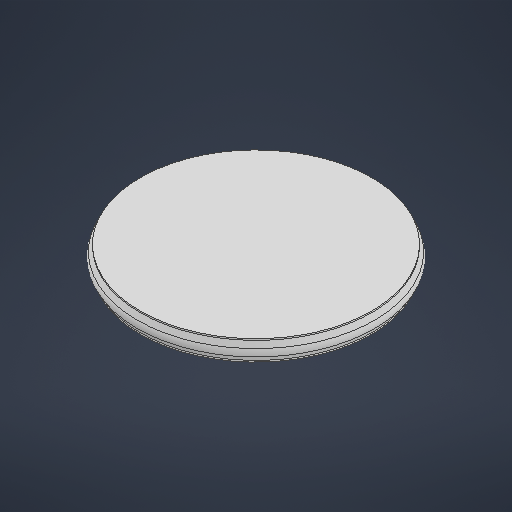
# Autodesk Inventor part: Game-Piece
Saved by Autodesk Inventor 2025 (Build 290162010, 162A)
## iProperties
Created: 2025-10-23
Part Number: Game-Piece
Material: Generic
Document SubType Name: Modeling
Designer: FizzyApple12
Density: 1 g/cm^3
Appearance: Default
Author: FizzyApple12
Autodesk Inventor part; units mm, degrees
ref_plane "YZ Plane" through (0, 0, 0) normal (1, 0, 0) x (0, 1, 0)
ref_plane "XZ Plane" through (0, 0, 0) normal (0, 1, 0) x (-1, 0, 0)
ref_plane "XY Plane" through (0, 0, 0) normal (0, 0, 1) x (1, 0, 0)
sketch "Sketch1" plane through (0, 0, 0) normal (1, 0, 0) x (0, 1, 0)
  line L0 (2.8, 16) -> (0, 16)
  line L1 (0, 16) -> (0, -16)
  line L2 (0, -16) -> (2.8, -16)
  line L3 (2.8, -16) -> (2.8, 16)
  line L4 (2.4, 12.7) -> (0.4, 12.7)
  line L5 (0.4, 12.7) -> (0.4, -12.7)
  line L6 (0.4, -12.7) -> (2.4, -12.7)
  line L7 (2.4, -12.7) -> (2.4, 12.7)
  line L8 (0, 0) -> (2.8, 0)
  line L9 (0.2, 16) -> (1.4, 16.6928)
  line L10 (1.4, 16.6928) -> (2.6, 16)
  line L11 (1.4, 16.6928) -> (1.4, 12.7) construction
  point P0 (0.4, 0)
  point P1 (2.4, 0)
  dimension "d0" = 0.4
  dimension "d1" = 0.4
  dimension "d2" = 2
  dimension "d4" = 32
  dimension "d5" = 25.4
  dimension "d6" = 240
  dimension "d8" = 0.2
  dimension "d14" = 0.2
  constraints: 24 end point, 4 midpoint, 4 parallel, 3 perpendicular, 3 point on line, 2 horizontal, 1 coincident
  measures "d0" distance between parallel lines of L1 L5
  measures "d1" distance between parallel lines of L3 L7
  measures "d2" distance between parallel lines of L7 L5
  measures "d4" distance between parallel lines of L2 L0
  measures "d5" distance between parallel lines of L6 L4
  measures "d8" distance of L0.start L10.end
  measures "d14" distance from line of L1 L9.start
revolve "Revolution1" add sketch "Sketch1" angle 360 about axis through (0, 0, 0) along (0, 1, 0) contours L3 L8 L7 L4 L5 L1 L0 | L0 L9 L10
chamfer "Chamfer1" [suppressed]
fillet "Fillet1" radius 1 1 edges at (0, 1.4, -16.6928)
equation "\"d14\" = d8"
body "Solid1"
